Autodesk Fusion 360 part; units mm, degrees
(part 2 of 3)
sketch "motor_base_geometry" plane through (0, 0, 0) normal (0, 1, 0) x (1, 0, 0)
  line L0 (0, 120) -> (0, 140)
  line L1 (0, -20) -> (0, 0)
  line L2 (0, 40) -> (0, 60)
  line L3 (0, 100) -> (0, 120)
  line L4 (0, 20) -> (0, 40)
  line L5 (0, 0) -> (0, 20)
  line L6 (0, -40) -> (0, -20)
  line L7 (0, -80) -> (0, -60)
  line L8 (5, -200) -> (5, -220)
  line L9 (5, -180) -> (5, -200)
  line L10 (5, -340) -> (5, -360)
  line L11 (0, -380) -> (0, -360)
  line L12 (5, -440) -> (5, -460)
  line L13 (0, -200) -> (0, -180)
  line L14 (5, -80) -> (5, -100)
  line L15 (6, -520) -> (6, 520)
  line L16 (5, 520) -> (5, 500)
  line L17 (0, -400) -> (0, -380)
  line L18 (5, 380) -> (5, 360)
  line L19 (0, -100) -> (0, -80)
  line L20 (0, -220) -> (0, -200)
  line L21 (5, 0) -> (5, -20)
  line L22 (5, -100) -> (5, -120)
  line L23 (0, -180) -> (0, -160)
  line L24 (5, 360) -> (5, 340)
  line L25 (0, -624) -> (0, -520)
  line L26 (5, -480) -> (5, -500)
  line L27 (5, 500) -> (5, 480)
  line L28 (0, -520) -> (5, -520)
  line L29 (0, -120) -> (0, -100)
  line L30 (0, -440) -> (0, -420)
  line L31 (0, -260) -> (0, -240)
  line L32 (5, -60) -> (5, -80)
  line L33 (5, 20) -> (5, 0)
  line L34 (5, -40) -> (5, -60)
  line L35 (5, 120) -> (5, 100)
  line L36 (5, 440) -> (5, 420)
  line L37 (5, 240) -> (5, 220)
  line L38 (6, 520) -> (5, 520)
  line L39 (5, -400) -> (5, -420)
  line L40 (0, -500) -> (0, -480)
  line L41 (5, -240) -> (5, -260)
  line L42 (5, 100) -> (5, 80)
  line L43 (5, 300) -> (5, 280)
  line L44 (5, -420) -> (5, -440)
  line L45 (5, -20) -> (5, -40)
  line L46 (0, -420) -> (0, -400)
  line L47 (0, 520) -> (0, 624)
  line L48 (0, -340) -> (0, -320)
  line L49 (5, -260) -> (5, -280)
  line L50 (0, -140) -> (0, -120)
  line L51 (5, 280) -> (5, 260)
  line L52 (0, -480) -> (0, -460)
  line L53 (5, 60) -> (5, 40)
  line L54 (5, -160) -> (5, -180)
  line L55 (5, 160) -> (5, 140)
  line L56 (5, 180) -> (5, 160)
  line L57 (5, 200) -> (5, 180)
  line L58 (5, 40) -> (5, 20)
  line L59 (5, 140) -> (5, 120)
  line L60 (0, 460) -> (0, 480)
  line L61 (26.7, -624) -> (0, -624)
  line L62 (0, 480) -> (0, 500)
  line L63 (5, 260) -> (5, 240)
  line L64 (5, 420) -> (5, 400)
  line L65 (5, 80) -> (5, 60)
  line L66 (5, 220) -> (5, 200)
  line L67 (5, -520) -> (6, -520)
  line L68 (5, 320) -> (5, 300)
  line L69 (5, 460) -> (5, 440)
  line L70 (5, 400) -> (5, 380)
  line L71 (5, 480) -> (5, 460)
  line L72 (5, 340) -> (5, 320)
  line L73 (0, -160) -> (0, -140)
  line L74 (5, -360) -> (5, -380)
  line L75 (0, -320) -> (0, -300)
  line L76 (5, -380) -> (5, -400)
  line L77 (5, -500) -> (0, -500)
  line L78 (0, -360) -> (0, -340)
  line L79 (5, -300) -> (5, -320)
  line L80 (5, -140) -> (5, -160)
  line L81 (0, -300) -> (0, -280)
  line L82 (0, -240) -> (0, -220)
  line L83 (5, -120) -> (5, -140)
  line L84 (26.7, 624) -> (26.7, -624)
  line L85 (0, 320) -> (0, 340)
  line L86 (0, 420) -> (0, 440)
  line L87 (0, -280) -> (0, -260)
  line L88 (5, -220) -> (5, -240)
  line L89 (0, -460) -> (0, -440)
  line L90 (5, -320) -> (5, -340)
  line L91 (5, -280) -> (5, -300)
  line L92 (5, -460) -> (5, -480)
  line L93 (0, 440) -> (0, 460)
  line L94 (0, 360) -> (0, 380)
  line L95 (0, 624) -> (26.7, 624)
  line L96 (0, 340) -> (0, 360)
  line L97 (0, 300) -> (0, 320)
  line L98 (0, 260) -> (0, 280)
  line L99 (0, 220) -> (0, 240)
  line L100 (0, 240) -> (0, 260)
  line L101 (0, 180) -> (0, 200)
  line L102 (0, 160) -> (0, 180)
  line L103 (0, 280) -> (0, 300)
  line L104 (0, 200) -> (0, 220)
  line L105 (0, 140) -> (0, 160)
  line L106 (0, 80) -> (0, 100)
  line L107 (0, 60) -> (0, 80)
  line L108 (0, -60) -> (0, -40)
  line L109 (0, 400) -> (0, 420)
  line L110 (0, 500) -> (0, 520)
  line L111 (0, 380) -> (0, 400)
  line L112 (7.5, -30) -> (7.5, -25.1667)
  line L113 (7.5, -25.1667) -> (10.5, -25.1667)
  line L114 (10.5, -30) -> (7.5, -30)
  line L115 (10.5, -25.1667) -> (10.5, -30)
  line L116 (7.5, -18.3333) -> (10.5, -18.3333)
  line L117 (10.5, -23.1667) -> (7.5, -23.1667)
  line L118 (10.5, -18.3333) -> (10.5, -23.1667)
  line L119 (7.5, -23.1667) -> (7.5, -18.3333)
  line L120 (7.5, -16.3333) -> (7.5, -11.5)
  line L121 (10.5, -11.5) -> (10.5, -16.3333)
  line L122 (10.5, -16.3333) -> (7.5, -16.3333)
  line L123 (7.5, -11.5) -> (10.5, -11.5)
  line L124 (10.5, -9.5) -> (7.5, -9.5)
  line L125 (7.5, -9.5) -> (7.5, -4.6667)
  line L126 (7.5, -4.6667) -> (10.5, -4.6667)
  line L127 (10.5, -4.6667) -> (10.5, -9.5)
  line L128 (7.5, 2.1667) -> (10.5, 2.1667)
  line L129 (10.5, 2.1667) -> (10.5, -2.6667)
  line L130 (10.5, -2.6667) -> (7.5, -2.6667)
  line L131 (7.5, -2.6667) -> (7.5, 2.1667)
  line L132 (10.5, 9) -> (10.5, 4.1667)
  line L133 (7.5, 4.1667) -> (7.5, 9)
  line L134 (7.5, 9) -> (10.5, 9)
  line L135 (10.5, 4.1667) -> (7.5, 4.1667)
  line L136 (10.5, 11) -> (7.5, 11)
  line L137 (7.5, 11) -> (7.5, 15.8333)
  line L138 (10.5, 15.8333) -> (10.5, 11)
  line L139 (7.5, 15.8333) -> (10.5, 15.8333)
  line L140 (7.5, 22.6667) -> (10.5, 22.6667)
  line L141 (10.5, 22.6667) -> (10.5, 17.8333)
  line L142 (7.5, 17.8333) -> (7.5, 22.6667)
  line L143 (10.5, 17.8333) -> (7.5, 17.8333)
  line L144 (10.5, 24.6667) -> (7.5, 24.6667)
  line L145 (7.5, 24.6667) -> (7.5, 29.5)
  line L146 (7.5, 29.5) -> (10.5, 29.5)
  line L147 (10.5, 29.5) -> (10.5, 24.6667)
  line L148 (10.5, 31.5) -> (7.5, 31.5)
  line L149 (7.5, 36.3333) -> (10.5, 36.3333)
  line L150 (7.5, 31.5) -> (7.5, 36.3333)
  line L151 (10.5, 36.3333) -> (10.5, 31.5)
  line L152 (7.5, 38.3333) -> (7.5, 43.1667)
  line L153 (10.5, 43.1667) -> (10.5, 38.3333)
  line L154 (7.5, 43.1667) -> (10.5, 43.1667)
  line L155 (10.5, 38.3333) -> (7.5, 38.3333)
  line L156 (10.5, 45.1667) -> (7.5, 45.1667)
  line L157 (7.5, 50) -> (10.5, 50)
  line L158 (10.5, 50) -> (10.5, 45.1667)
  line L159 (7.5, 45.1667) -> (7.5, 50)
  line L160 (10.5, 45.1667) -> (10.5, 43.1667)
  line L161 (10.5, 38.3333) -> (10.5, 36.3333)
  line L162 (10.5, 31.5) -> (10.5, 29.5)
  line L163 (10.5, 24.6667) -> (10.5, 22.6667)
  line L164 (10.5, 17.8333) -> (10.5, 15.8333)
  line L165 (10.5, 4.1667) -> (10.5, 2.1667)
  line L166 (10.5, -2.6667) -> (10.5, -4.6667)
  line L167 (10.5, -9.5) -> (10.5, -11.5)
  line L168 (10.5, -16.3333) -> (10.5, -18.3333)
  line L169 (10.5, -23.1667) -> (10.5, -25.1667)
  line L170 (17.8, 45.25) -> (12.3, 45.25)
  line L171 (17.8, 47.25) -> (12.3, 47.25)
  line L172 (12.3, 44.75) -> (17.8, 44.75)
  line L173 (17.8, 39.25) -> (12.3, 39.25)
  line L174 (17.8, 37.25) -> (12.3, 37.25)
  line L175 (17.8, 30.75) -> (17.8, 31.25)
  line L176 (17.8, 26.75) -> (17.8, 27.25)
  line L177 (17.8, 40.75) -> (17.8, 41.25)
  line L178 (12.3, 35.25) -> (12.3, 36.75)
  line L179 (17.8, 36.75) -> (17.8, 37.25)
  line L180 (17.8, 28.75) -> (17.8, 29.25)
  line L181 (12.3, 28.75) -> (17.8, 28.75)
  line L182 (12.3, 40.75) -> (17.8, 40.75)
  line L183 (12.3, 38.75) -> (17.8, 38.75)
  line L184 (17.8, 41.25) -> (12.3, 41.25)
  line L185 (12.3, 33.25) -> (12.3, 34.75)
  line L186 (17.8, 29.25) -> (12.3, 29.25)
  line L187 (17.8, 49.25) -> (12.3, 49.25)
  line L188 (17.8, 25.25) -> (12.3, 25.25)
  line L189 (17.8, 35.25) -> (12.3, 35.25)
  line L190 (17.8, 38.75) -> (17.8, 39.25)
  line L191 (12.3, 39.25) -> (12.3, 40.75)
  line L192 (17.8, 34.75) -> (17.8, 35.25)
  line L193 (12.3, 42.75) -> (17.8, 42.75)
  line L194 (12.3, 27.25) -> (12.3, 28.75)
  line L195 (17.8, 48.75) -> (17.8, 49.25)
  line L196 (12.3, 36.75) -> (17.8, 36.75)
  line L197 (17.8, 43.25) -> (12.3, 43.25)
  line L198 (17.8, 46.75) -> (17.8, 47.25)
  line L199 (12.3, 49.25) -> (12.3, 50.75)
  line L200 (12.3, 47.25) -> (12.3, 48.75)
  line L201 (12.3, 30.75) -> (17.8, 30.75)
  line L202 (12.3, 29.25) -> (12.3, 30.75)
  line L203 (12.3, 37.25) -> (12.3, 38.75)
  line L204 (12.3, 43.25) -> (12.3, 44.75)
  line L205 (17.8, 50.75) -> (17.8, 51.25)
  line L206 (12.3, 50.75) -> (17.8, 50.75)
  line L207 (12.3, 25.25) -> (12.3, 26.75)
  line L208 (12.3, 46.75) -> (17.8, 46.75)
  line L209 (17.8, 31.25) -> (12.3, 31.25)
  line L210 (17.8, -9.25) -> (17.8, -8.75)
  line L211 (12.3, 3.25) -> (12.3, 4.75)
  line L212 (12.3, 24.75) -> (17.8, 24.75)
  line L213 (17.8, -7.25) -> (17.8, -6.75)
  line L214 (17.8, 12.75) -> (17.8, 13.25)
  line L215 (17.8, 16.75) -> (17.8, 17.25)
  line L216 (17.8, 15.25) -> (12.3, 15.25)
  line L217 (12.3, 2.75) -> (17.8, 2.75)
  line L218 (17.8, -6.75) -> (12.3, -6.75)
  line L219 (17.8, -2.75) -> (12.3, -2.75)
  line L220 (12.3, 10.75) -> (17.8, 10.75)
  line L221 (17.8, 21.25) -> (12.3, 21.25)
  line L222 (12.3, 22.75) -> (17.8, 22.75)
  line L223 (12.3, 1.25) -> (12.3, 2.75)
  line L224 (17.8, 32.75) -> (17.8, 33.25)
  line L225 (12.3, 41.25) -> (12.3, 42.75)
  line L226 (17.8, 24.75) -> (17.8, 25.25)
  line L227 (17.8, 19.25) -> (12.3, 19.25)
  line L228 (12.3, 26.75) -> (17.8, 26.75)
  line L229 (12.3, 45.25) -> (12.3, 46.75)
  line L230 (17.8, 6.75) -> (17.8, 7.25)
  line L231 (12.3, 48.75) -> (17.8, 48.75)
  line L232 (17.8, 51.25) -> (17.8, 51.4522)
  line L233 (11.5, 51.4522) -> (11.5, 51.25)
  line L234 (11.5, 51.25) -> (11.5, 50)
  line L235 (17.8, 8.75) -> (17.8, 9.25)
  line L236 (12.3, 31.25) -> (12.3, 32.75)
  line L237 (17.8, 33.25) -> (12.3, 33.25)
  line L238 (12.3, -1.25) -> (17.8, -1.25)
  line L239 (17.8, 27.25) -> (12.3, 27.25)
  line L240 (17.8, -17.25) -> (17.8, -16.75)
  line L241 (17.8, 51.4522) -> (11.5, 51.4522)
  line L242 (17.8, -31.25) -> (17.8, -30.75)
  line L243 (17.8, -26.75) -> (12.3, -26.75)
  line L244 (12.3, 32.75) -> (17.8, 32.75)
  line L245 (17.8, 9.25) -> (12.3, 9.25)
  line L246 (12.3, -3.25) -> (17.8, -3.25)
  line L247 (17.8, 10.75) -> (17.8, 11.25)
  line L248 (12.3, 15.25) -> (12.3, 16.75)
  line L249 (12.3, -6.75) -> (12.3, -5.25)
  line L250 (12.3, 12.75) -> (17.8, 12.75)
  line L251 (12.3, 6.75) -> (17.8, 6.75)
  line L252 (17.8, 22.75) -> (17.8, 23.25)
  line L253 (17.8, -4.75) -> (12.3, -4.75)
  line L254 (12.3, -0.75) -> (12.3, 0.75)
  line L255 (11.5, 50) -> (11.5, -30)
  line L256 (17.8, -24.75) -> (12.3, -24.75)
  line L257 (17.8, -12.75) -> (12.3, -12.75)
  line L258 (17.8, -29.25) -> (17.8, -28.75)
  line L259 (17.8, -28.75) -> (12.3, -28.75)
  line L260 (17.8, -16.75) -> (12.3, -16.75)
  line L261 (12.3, -29.25) -> (17.8, -29.25)
  line L262 (12.3, -25.25) -> (17.8, -25.25)
  line L263 (12.3, -16.75) -> (12.3, -15.25)
  line L264 (17.8, -23.25) -> (17.8, -22.75)
  line L265 (17.8, 44.75) -> (17.8, 45.25)
  line L266 (17.8, -10.75) -> (12.3, -10.75)
  line L267 (9, -35) -> (6.5, -35)
  line L268 (12.3, -32.75) -> (12.3, -31.25)
  line L269 (12.3, -22.75) -> (12.3, -21.25)
  line L270 (12.3, -18.75) -> (12.3, -17.25)
  line L271 (17.8, -30.75) -> (12.3, -30.75)
  line L272 (12.3, -15.25) -> (17.8, -15.25)
  line L273 (17.8, -25.25) -> (17.8, -24.75)
  line L274 (17.8, -15.25) -> (17.8, -14.75)
  line L275 (12.3, -12.75) -> (12.3, -11.25)
  line L276 (10.7, -35) -> (9, -35)
  line L277 (17.8, -38) -> (17.8, -33.25)
  line L278 (12.3, -23.25) -> (17.8, -23.25)
  line L279 (17.8, -32.75) -> (12.3, -32.75)
  line L280 (17.8, -21.25) -> (17.8, -20.75)
  line L281 (6.5, -35) -> (6.5, -38)
  line L282 (12.3, -28.75) -> (12.3, -27.25)
  line L283 (12.3, -27.25) -> (17.8, -27.25)
  line L284 (17.8, -11.25) -> (17.8, -10.75)
  line L285 (12.3, 34.75) -> (17.8, 34.75)
  line L286 (12.3, -14.75) -> (12.3, -13.25)
  line L287 (12.3, -21.25) -> (17.8, -21.25)
  line L288 (11.5, -30) -> (11.5, -35)
  line L289 (12.3, -19.25) -> (17.8, -19.25)
  line L290 (17.8, -14.75) -> (12.3, -14.75)
  line L291 (17.8, -18.75) -> (12.3, -18.75)
  line L292 (12.3, 13.25) -> (12.3, 14.75)
  line L293 (12.3, 11.25) -> (12.3, 12.75)
  line L294 (12.3, -4.75) -> (12.3, -3.25)
  line L295 (17.8, 0.75) -> (17.8, 1.25)
  line L296 (12.3, 16.75) -> (17.8, 16.75)
  line L297 (17.8, 11.25) -> (12.3, 11.25)
  line L298 (17.8, -13.25) -> (17.8, -12.75)
  line L299 (17.8, -22.75) -> (12.3, -22.75)
  line L300 (17.8, -33.25) -> (17.8, -32.75)
  line L301 (11.5, -35) -> (10.7, -35)
  line L302 (12.3, -8.75) -> (12.3, -7.25)
  line L303 (12.3, -17.25) -> (17.8, -17.25)
  line L304 (12.3, -11.25) -> (17.8, -11.25)
  line L305 (17.8, 42.75) -> (17.8, 43.25)
  line L306 (6.5, -38) -> (17.8, -38)
  line L307 (12.3, -20.75) -> (12.3, -19.25)
  line L308 (17.8, -27.25) -> (17.8, -26.75)
  line L309 (17.8, -19.25) -> (17.8, -18.75)
  line L310 (12.3, -31.25) -> (17.8, -31.25)
  line L311 (17.8, -20.75) -> (12.3, -20.75)
  line L312 (12.3, -9.25) -> (17.8, -9.25)
  line L313 (12.3, -30.75) -> (12.3, -29.25)
  line L314 (12.3, -13.25) -> (17.8, -13.25)
  line L315 (17.8, -8.75) -> (12.3, -8.75)
  line L316 (12.3, -7.25) -> (17.8, -7.25)
  line L317 (12.3, -26.75) -> (12.3, -25.25)
  line L318 (12.3, -24.75) -> (12.3, -23.25)
  line L319 (12.3, -10.75) -> (12.3, -9.25)
  line L320 (12.3, 17.25) -> (12.3, 18.75)
  line L321 (17.8, 17.25) -> (12.3, 17.25)
  line L322 (12.3, 20.75) -> (17.8, 20.75)
  line L323 (17.8, -1.25) -> (17.8, -0.75)
  line L324 (17.8, 13.25) -> (12.3, 13.25)
  line L325 (17.8, -0.75) -> (12.3, -0.75)
  line L326 (17.8, -5.25) -> (17.8, -4.75)
  line L327 (17.8, 3.25) -> (12.3, 3.25)
  line L328 (17.8, 5.25) -> (12.3, 5.25)
  line L329 (17.8, 2.75) -> (17.8, 3.25)
  line L330 (17.8, 20.75) -> (17.8, 21.25)
  line L331 (17.8, 1.25) -> (12.3, 1.25)
  line L332 (12.3, 23.25) -> (12.3, 24.75)
  line L333 (12.3, 4.75) -> (17.8, 4.75)
  line L334 (12.3, 7.25) -> (12.3, 8.75)
  line L335 (12.3, 18.75) -> (17.8, 18.75)
  line L336 (12.3, -2.75) -> (12.3, -1.25)
  line L337 (17.8, 18.75) -> (17.8, 19.25)
  line L338 (12.3, 0.75) -> (17.8, 0.75)
  line L339 (17.8, 4.75) -> (17.8, 5.25)
  line L340 (12.3, 21.25) -> (12.3, 22.75)
  line L341 (17.8, 14.75) -> (17.8, 15.25)
  line L342 (17.8, -3.25) -> (17.8, -2.75)
  line L343 (17.8, 23.25) -> (12.3, 23.25)
  line L344 (12.3, 14.75) -> (17.8, 14.75)
  line L345 (12.3, -5.25) -> (17.8, -5.25)
  line L346 (12.3, 9.25) -> (12.3, 10.75)
  line L347 (12.3, 19.25) -> (12.3, 20.75)
  line L348 (12.3, 5.25) -> (12.3, 6.75)
  line L349 (12.3, 8.75) -> (17.8, 8.75)
  line L350 (17.8, 7.25) -> (12.3, 7.25)
  line L351 (6.5, -35) -> (6.5, 55)
  line L352 (0, -520) -> (0, -500)
  line L353 (5, -500) -> (5, -520)
  line L354 (0, -480) -> (5, -480)
  line L355 (0, -460) -> (5, -460)
  line L356 (0, -440) -> (5, -440)
  line L357 (0, -420) -> (5, -420)
  line L358 (0, -400) -> (5, -400)
  line L359 (0, -380) -> (5, -380)
  line L360 (0, -360) -> (5, -360)
  line L361 (0, -340) -> (5, -340)
  line L362 (0, -320) -> (5, -320)
  line L363 (0, -300) -> (5, -300)
  line L364 (0, -280) -> (5, -280)
  line L365 (0, -260) -> (5, -260)
  line L366 (0, -240) -> (5, -240)
  line L367 (0, -220) -> (5, -220)
  line L368 (0, -200) -> (5, -200)
  line L369 (0, -180) -> (5, -180)
  line L370 (0, -160) -> (5, -160)
  line L371 (0, -140) -> (5, -140)
  line L372 (0, -120) -> (5, -120)
  line L373 (0, -100) -> (5, -100)
  line L374 (0, -80) -> (5, -80)
  line L375 (0, -60) -> (5, -60)
  line L376 (0, -40) -> (5, -40)
  line L377 (0, -20) -> (5, -20)
  line L378 (0, 0) -> (5, 0)
  line L379 (0, 20) -> (5, 20)
  line L380 (0, 40) -> (5, 40)
  line L381 (0, 60) -> (5, 60)
  line L382 (0, 80) -> (5, 80)
  line L383 (0, 100) -> (5, 100)
  line L384 (0, 120) -> (5, 120)
  line L385 (0, 140) -> (5, 140)
  line L386 (0, 160) -> (5, 160)
  line L387 (0, 180) -> (5, 180)
  line L388 (0, 200) -> (5, 200)
  line L389 (0, 220) -> (5, 220)
  line L390 (0, 240) -> (5, 240)
  line L391 (0, 260) -> (5, 260)
  line L392 (0, 280) -> (5, 280)
  line L393 (0, 300) -> (5, 300)
  line L394 (0, 320) -> (5, 320)
  line L395 (0, 340) -> (5, 340)
  line L396 (0, 360) -> (5, 360)
  line L397 (0, 380) -> (5, 380)
  line L398 (0, 400) -> (5, 400)
  line L399 (0, 420) -> (5, 420)
  line L400 (0, 440) -> (5, 440)
  line L401 (0, 460) -> (5, 460)
  line L402 (0, 480) -> (5, 480)
  line L403 (0, 500) -> (5, 500)
  line L404 (0, 520) -> (5, 520)
  line L405 (17.8, -33.25) -> (12.3, -33.25)
  line L406 (12.3, -33.25) -> (12.3, -34.75)
  line L407 (10.5, 11) -> (10.5, 9)
  line L408 (12.3, -34.75) -> (12.3, -35)
  line L409 (12.3, -35) -> (11.5, -35)
  line L410 (9, -35) -> (9.1, -35)
  line L411 (12.3, -35) -> (12.4, -35)
  line L412 (12.4, -35) -> (12.4, -33.25)
  line L413 (10.5, 50) -> (11.4, 50)
  line L414 (11.4, 50) -> (11.4, 51.4522)
  line L415 (11.4, 51.4522) -> (11.5, 51.4522)
  line L416 (6.5, 55) -> (17.8, 55)
  line L417 (17.8, 55) -> (17.8, 51.4522)
  line L418 (10.5, -30) -> (10.7, -30)
  line L419 (10.7, -30) -> (10.7, -33)
  line L420 (10.7, -33) -> (10.7, -35)
revolve "Revolve1" add sketch "motor_base_geometry" angle 360 about axis through (0, 0, 20) along (0, 0, -1) contours L112 L113 L114 L115
chamfer "Chamfer1" distance 0.2 angle 45 4 edges at (-9.7894, -3.797, 30) (-9.7894, -3.797, 25.1667) (-6.9925, -2.7121, 30) (-6.9925, -2.7121, 25.1667)
named bodies: "coil"

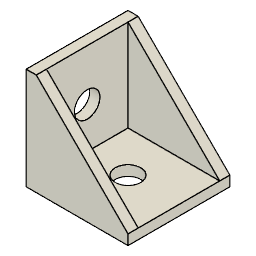
design "Aluminium connections"
Autodesk Fusion 360 part; units mm, degrees
sketch "Base & hole" plane through (0, 0, 0) normal (0, 1, 0) x (1, 0, 0)
  line L0 (0, 0) -> (20, 0)
  line L1 (20, 0) -> (20, 20)
  line L2 (20, 20) -> (0, 20)
  line L3 (0, 20) -> (0, 0)
  circle A0 centre (10, 10) radius 2.5
  dimension "d1" = 20
  dimension "d2" = 20
  dimension "d3" = 5
  constraint horizontal L0
  constraint vertical L1
  constraint horizontal L2
  constraint vertical L3
  constraint coincident L0.start L3.end
  measures "d1" distance of L0.start L0.end
  measures "d2" distance of L0.start L2.end
  measures "d3" diameter of A0
extrude "Extrude1" add sketch "Base & hole" along normal blind 20
sketch "Top" plane through (0, 20, 0) normal (0, 1, 0) x (-1, 0, 0)
  circle A0 centre (-10, -10) radius 2.5
  line L0 (0, -20) -> (0, 0)
  line L1 (0, 0) -> (-20, 0)
  line L2 (-20, 0) -> (-20, -20)
  line L3 (-20, -20) -> (0, -20)
  line L4 (-20, -20) -> (-20, -18) construction
  line L5 (-20, -18) -> (-2, -18)
  line L6 (-2, -18) -> (-2, -2)
  line L7 (-2, -2) -> (-20, -2)
  dimension "d6" = 2
  dimension "d7" = 18
  dimension "d8" = 16
  constraint coincident L2.end L3.start
  constraint perpendicular L3 L4
  constraint perpendicular L0 L5
  constraint perpendicular L3 L6
  constraint coincident L2 L7.end
  constraint perpendicular L2 L7
  measures "d6" distance of L2.end L4.end
  measures "d7" distance of L4.end L5.end
  measures "d8" distance of L5.end L6.end
extrude "Extrude2" cut sketch "Top" against normal blind 18 contours L2 L5 L6 L7
sketch "Side removal" plane through (0, 0, 0) normal (0, 0, 1) x (1, 0, 0)
  line L0 (0, 0) -> (20, 0)
  line L1 (20, 0) -> (20, 20)
  line L2 (20, 20) -> (0, 20)
  line L3 (0, 20) -> (0, 0)
  line L4 (0, 20) -> (2, 20)
  line L5 (20, 0) -> (20, 2)
  line L6 (20, 2) -> (2, 20)
  dimension "d11" = 2
  dimension "d12" = 2
  constraint coincident L2.end L3.start
  constraint perpendicular L3 L4
  constraint coincident L0.end L1.start
  constraint perpendicular L0 L5
  measures "d11" distance of L2.end L4.end
  measures "d12" distance of L0.end L5.end
extrude "Extrude3" cut sketch "Side removal" against normal blind 30 contours L1 L2 L6
sketch "side hole" plane through (0, 0, 0) normal (-1, 0, 0) x (0, 0, 1)
  line L0 (-20, 0) -> (0, 0)
  line L1 (0, 0) -> (0, 20)
  line L2 (0, 20) -> (-20, 20)
  line L3 (-20, 20) -> (-20, 0)
  circle A0 centre (-10, 10) radius 2.5
  dimension "d15" = 5
  measures "d15" diameter of A0
extrude "Extrude4" cut sketch "side hole" against normal blind 5 contours A0

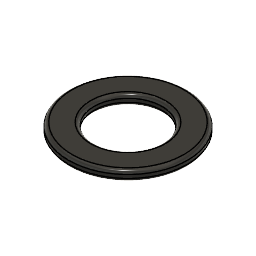
design "m2 by 0.3 spacer"
Autodesk Fusion 360 part; units mm, degrees
sketch "Sketch1" plane through (0, 0, 0) normal (0, 1, 0) x (1, 0, 0)
  circle A0 centre (0, 0) radius 1
  circle A1 centre (0, 0) radius 1.75
  dimension "d1" = 2
  dimension "d2" = 3.5
  constraint coincident A0.centre A1.centre
  measures "d1" diameter of A0
  measures "d2" diameter of A1
extrude "Extrude1" add sketch "Sketch1" along normal blind 0.3
fillet "Fillet1" radius 0.1 4 edges at (-0.9323, 0.3, -0.3616) (-0.9323, 0, -0.3616) (-1.6316, 0.3, 0.6328) (-1.6316, 0, 0.6328)

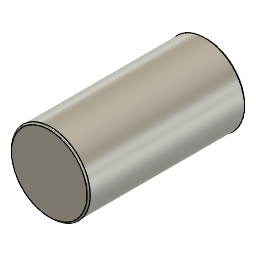
design "15mm by 20mm axial magnet"
Autodesk Fusion 360 part; units mm, degrees
sketch "Sketch1" plane through (0, 0, 0) normal (0, 0, 1) x (1, 0, 0)
  circle A0 centre (0, 0) radius 5
  dimension "d1" = 10
  constraint coincident A0.centre origin
  measures "d1" diameter of A0
extrude "Extrude1" add sketch "Sketch1" along normal blind 20
fillet "Fillet1" radius 0.2 2 edges at (-4.6616, -1.8081, 20) (-4.6616, -1.8081, 0)

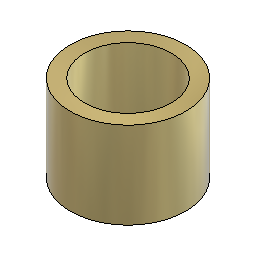
design "M3 x 3 Insert"
Autodesk Fusion 360 part; units mm, degrees
sketch "Sketch1" plane through (0, 0, 0) normal (0, 1, 0) x (1, 0, 0)
  circle A0 centre (0, 0) radius 1.5
  circle A1 centre (0, 0) radius 2
  dimension "d1" = 3
  dimension "d2" = 4
  constraint coincident A0.centre A1.centre
  measures "d1" diameter of A0
  measures "d2" diameter of A1
extrude "Extrude1" add sketch "Sketch1" along normal blind 5
extrude "Extrude2" cut 1 faces at (1.8259, 5, 0.0994) along direction (0, -1, 0) blind 2

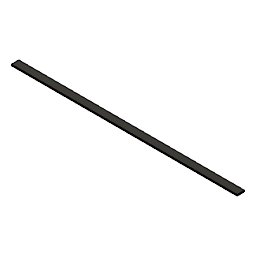
design "linear scale"
Autodesk Fusion 360 part; units mm, degrees
sketch "base" plane through (0, 0, 0) normal (0, 1, 0) x (1, 0, 0)
  line L0 (0, 0) -> (-300, 0)
  line L1 (-300, 0) -> (-300, 10)
  line L2 (-300, 10) -> (0, 10)
  line L3 (0, 10) -> (0, 0)
  dimension "d1" = 300
  dimension "d2" = 10
  constraint coincident L0.start L3.end
  constraint horizontal L0
  constraint perpendicular L0 L1
  constraint perpendicular L1 L2
  constraint perpendicular L0 L3
  measures "d1" distance of L0.start L0.end
  measures "d2" distance of L0.end L1.end
extrude "Extrude1" add sketch "base" along normal blind 1.4
named bodies: "main"

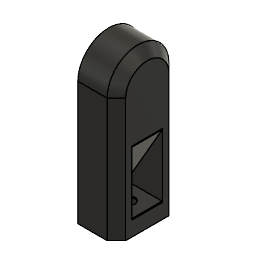
design "stator_holders"
Autodesk Fusion 360 part; units mm, degrees
sketch "Base" plane through (0, 0, 0) normal (1, 0, 0) x (0, 0, -1)
  circle A0 centre (0, 0) radius 6.1
  circle A1 centre (0, 0) radius 10 construction
  line L0 (0, 0) -> (-10, 0) construction
  line L1 (0, 0) -> (0, -40) construction
  line L2 (0, -40) -> (-10, -40)
  line L3 (-10, -40) -> (-10, 0)
  line L4 (10, -40) -> (10, 0)
  line L5 (0, -40) -> (10, -40)
  line L6 (0, 0) -> (0, 10) construction
  arc A2 (10, 0) -> (-10, 0) centre (0, 0) ccw
  dimension "d1" = 12.2
  dimension "d2" = 20
  dimension "d3" = 40
  dimension "d4" = 10
  constraint coincident A0.centre A1.centre
  constraint concentric A0 A1
  constraint coincident A1 L0.end
  constraint horizontal L0
  constraint perpendicular L0 L1
  constraint perpendicular L1 L2
  constraint symmetric L0.end L1 L4.end
  constraint symmetric L2.start L1 L5.start
  constraint symmetric L1 L2.end L4.start
  constraint coincident A1 L6.end
  constraint perpendicular L0 L6
  constraint coincident L6.end A2
  measures "d1" diameter of A0
  measures "d2" diameter of A1
  measures "d3" distance of A0.centre L1.end
  measures "d4" distance of L1.end L2.end
extrude "Extrude1" add sketch "Base" along normal blind 12.5 contours A0 | L2 L3 L4 L5 A2
extrude "Extrude2" cut sketch "Base" along normal blind 10 contours A0
chamfer "Chamfer1" distance 3 angle 45 3 edges at (12.5, 10, 0) (12.5, -20, 10) (12.5, -20, -10)
ref_plane "WorkPlane1" through (6.25, -20, 0) normal (0, 0, -1) x (0, 1, 0)
sketch "Bolt" plane through (0, 0, 0) normal (0, 0, -1) x (0, 1, 0)
  line L0 (0, 0) -> (-30, 0) construction
  line L1 (-30, 0) -> (-30, 12.5) construction
  line L2 (-30, 12.5) -> (0, 12.5) construction
  line L3 (0, 12.5) -> (0, 0) construction
  line L4 (-30, 12.5) -> (-35, 12.5) construction
  line L5 (-35, 12.5) -> (-35, 0) construction
  line L6 (-35, 12.5) -> (-35, 2.5)
  line L7 (-35, 2.5) -> (-32, 2.5)
  line L8 (-32, 2.5) -> (-14.6795, 12.5)
  line L9 (-35, 12.5) -> (-14.6795, 12.5)
  dimension "d11" = 12.5
  dimension "d12" = 10
  dimension "d13" = 20
  constraint horizontal L0
  constraint vertical L1
  constraint horizontal L2
  constraint vertical L3
  constraint coincident L0.start L3.end
  constraint coincident L2 L4.end
  constraint coincident L0 L5.end
  constraint perpendicular L0 L5
  constraint perpendicular L2 L6
  constraint perpendicular L6 L7
  constraint coincident L2 L8.end
  measures "d11" distance of L0.start L2.end
  measures "d12" distance of L4.end L6.end
  measures "d13" distance of L7.end L8.end
extrude "Extrude3" cut sketch "Bolt" along normal blind 5
extrude "Extrude4" cut 1 faces at (9.1667, -27.2265, 0) along direction (0, 0, 1) blind 5
sketch "Sketch3" plane through (0, -35, 0) normal (0, 1, 0) x (-1, 0, 0)
  line L0 (-12.5, 5) -> (-12.5, -5)
  line L1 (-12.5, -5) -> (-2.5, -5)
  line L2 (-2.5, -5) -> (-2.5, 5)
  line L3 (-2.5, 5) -> (-12.5, 5)
  line L4 (-12.5, 5) -> (-2.5, 5)
  line L5 (-2.5, 5) -> (-2.5, -5)
  line L6 (-2.5, -5) -> (-12.5, -5)
  line L7 (-12.5, -5) -> (-12.5, 5)
  circle A0 centre (-7, 0) radius 1.5
  dimension "d18" = 3
  constraint horizontal L4
  constraint vertical L5
  constraint horizontal L6
  constraint vertical L7
  constraint coincident L1.end L2.start
  constraint coincident L0.start L3.end
  measures "d18" diameter of A0
extrude "Extrude5" cut sketch "Sketch3" against normal blind 6 contours A0
chamfer "Chamfer2" distance 0.2 angle 45 1 edges at (8.3985, -35, 0.5424)
chamfer "Chamfer3" distance 0.2 angle 45 4 edges at (2.5, -35, 0) (2.5, -32, 0) (12.5, -14.6795, 0) (12.5, -35, 0)
chamfer "Chamfer4" distance 0.3 angle 45 1 edges at (0, -2.2059, 5.6872)

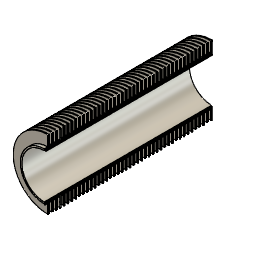
design "heat_sink"
Autodesk Fusion 360 part; units mm, degrees
sketch "motor_base_geometry" plane through (0, 0, 0) normal (0, 1, 0) x (1, 0, 0)
  line L0 (0, -624) -> (0, -520)
  line L1 (0, 624) -> (26.7, 624)
  line L2 (26.7, 624) -> (26.7, -624)
  line L3 (26.7, -624) -> (0, -624)
  line L4 (0, 520) -> (0, 624)
  line L5 (7.5, -30) -> (7.5, -25.1667)
  line L6 (7.5, -25.1667) -> (10.5, -25.1667)
  line L7 (10.5, -30) -> (7.5, -30)
  line L8 (7.5, -23.1667) -> (7.5, -18.3333)
  line L9 (7.5, -18.3333) -> (10.5, -18.3333)
  line L10 (10.5, -23.1667) -> (7.5, -23.1667)
  line L11 (7.5, -16.3333) -> (7.5, -11.5)
  line L12 (7.5, -11.5) -> (10.5, -11.5)
  line L13 (10.5, -16.3333) -> (7.5, -16.3333)
  line L14 (7.5, -9.5) -> (7.5, -4.6667)
  line L15 (7.5, -4.6667) -> (10.5, -4.6667)
  line L16 (10.5, -9.5) -> (7.5, -9.5)
  line L17 (7.5, -2.6667) -> (7.5, 2.1667)
  line L18 (7.5, 2.1667) -> (10.5, 2.1667)
  line L19 (10.5, -2.6667) -> (7.5, -2.6667)
  line L20 (7.5, 4.1667) -> (7.5, 9)
  line L21 (7.5, 9) -> (10.5, 9)
  line L22 (10.5, 4.1667) -> (7.5, 4.1667)
  line L23 (7.5, 11) -> (7.5, 15.8333)
  line L24 (7.5, 15.8333) -> (10.5, 15.8333)
  line L25 (10.5, 11) -> (7.5, 11)
  line L26 (7.5, 17.8333) -> (7.5, 22.6667)
  line L27 (7.5, 22.6667) -> (10.5, 22.6667)
  line L28 (10.5, 17.8333) -> (7.5, 17.8333)
  line L29 (7.5, 24.6667) -> (7.5, 29.5)
  line L30 (7.5, 29.5) -> (10.5, 29.5)
  line L31 (10.5, 24.6667) -> (7.5, 24.6667)
  line L32 (7.5, 31.5) -> (7.5, 36.3333)
  line L33 (7.5, 36.3333) -> (10.5, 36.3333)
  line L34 (10.5, 31.5) -> (7.5, 31.5)
  line L35 (7.5, 38.3333) -> (7.5, 43.1667)
  line L36 (7.5, 43.1667) -> (10.5, 43.1667)
  line L37 (10.5, 38.3333) -> (7.5, 38.3333)
  line L38 (7.5, 45.1667) -> (7.5, 50)
  line L39 (7.5, 50) -> (10.5, 50)
  line L40 (10.5, 45.1667) -> (7.5, 45.1667)
  line L41 (10.5, 45.1667) -> (10.5, 43.1667)
  line L42 (10.5, 38.3333) -> (10.5, 36.3333)
  line L43 (10.5, 31.5) -> (10.5, 29.5)
  line L44 (10.5, 24.6667) -> (10.5, 22.6667)
  line L45 (10.5, 17.8333) -> (10.5, 15.8333)
  line L46 (10.5, 4.1667) -> (10.5, 2.1667)
  line L47 (10.5, -2.6667) -> (10.5, -4.6667)
  line L48 (10.5, -9.5) -> (10.5, -11.5)
  line L49 (10.5, -16.3333) -> (10.5, -18.3333)
  line L50 (10.5, -23.1667) -> (10.5, -25.1667)
  line L51 (11.5, -30) -> (11.5, -35)
  line L52 (6.5, -35) -> (6.5, 55)
  line L53 (10.5, -25.1667) -> (10.5, -30)
  line L54 (10.5, -18.3333) -> (10.5, -23.1667)
  line L55 (10.5, -11.5) -> (10.5, -16.3333)
  line L56 (10.5, -4.6667) -> (10.5, -9.5)
  line L57 (10.5, 2.1667) -> (10.5, -2.6667)
  line L58 (10.5, 9) -> (10.5, 4.1667)
  line L59 (10.5, 15.8333) -> (10.5, 11)
  line L60 (10.5, 22.6667) -> (10.5, 17.8333)
  line L61 (10.5, 29.5) -> (10.5, 24.6667)
  line L62 (10.5, 36.3333) -> (10.5, 31.5)
  line L63 (10.5, 43.1667) -> (10.5, 38.3333)
  line L64 (10.5, 50) -> (10.5, 45.1667)
  line L65 (0, -520) -> (0, -500)
  line L66 (0, -500) -> (0, -480)
  line L67 (0, -500) -> (5, -500)
  line L68 (5, -500) -> (5, -520)
  line L69 (5, -520) -> (0, -520)
  line L70 (0, -480) -> (0, -460)
  line L71 (0, -480) -> (5, -480)
  line L72 (5, -480) -> (5, -500)
  line L73 (0, -460) -> (0, -440)
  line L74 (0, -460) -> (5, -460)
  line L75 (5, -460) -> (5, -480)
  line L76 (0, -440) -> (0, -420)
  line L77 (0, -440) -> (5, -440)
  line L78 (5, -440) -> (5, -460)
  line L79 (0, -420) -> (0, -400)
  line L80 (0, -420) -> (5, -420)
  line L81 (5, -420) -> (5, -440)
  line L82 (0, -400) -> (0, -380)
  line L83 (0, -400) -> (5, -400)
  line L84 (5, -400) -> (5, -420)
  line L85 (0, -380) -> (0, -360)
  line L86 (0, -380) -> (5, -380)
  line L87 (5, -380) -> (5, -400)
  line L88 (0, -360) -> (0, -340)
  line L89 (0, -360) -> (5, -360)
  line L90 (5, -360) -> (5, -380)
  line L91 (0, -340) -> (0, -320)
  line L92 (0, -340) -> (5, -340)
  line L93 (5, -340) -> (5, -360)
  line L94 (0, -320) -> (0, -300)
  line L95 (0, -320) -> (5, -320)
  line L96 (5, -320) -> (5, -340)
  line L97 (0, -300) -> (0, -280)
  line L98 (0, -300) -> (5, -300)
  line L99 (5, -300) -> (5, -320)
  line L100 (0, -280) -> (0, -260)
  line L101 (0, -280) -> (5, -280)
  line L102 (5, -280) -> (5, -300)
  line L103 (0, -260) -> (0, -240)
  line L104 (0, -260) -> (5, -260)
  line L105 (5, -260) -> (5, -280)
  line L106 (0, -240) -> (0, -220)
  line L107 (0, -240) -> (5, -240)
  line L108 (5, -240) -> (5, -260)
  line L109 (0, -220) -> (0, -200)
  line L110 (0, -220) -> (5, -220)
  line L111 (5, -220) -> (5, -240)
  line L112 (0, -200) -> (0, -180)
  line L113 (0, -200) -> (5, -200)
  line L114 (5, -200) -> (5, -220)
  line L115 (0, -180) -> (0, -160)
  line L116 (0, -180) -> (5, -180)
  line L117 (5, -180) -> (5, -200)
  line L118 (0, -160) -> (0, -140)
  line L119 (0, -160) -> (5, -160)
  line L120 (5, -160) -> (5, -180)
  line L121 (0, -140) -> (0, -120)
  line L122 (0, -140) -> (5, -140)
  line L123 (5, -140) -> (5, -160)
  line L124 (0, -120) -> (0, -100)
  line L125 (0, -120) -> (5, -120)
  line L126 (5, -120) -> (5, -140)
  line L127 (0, -100) -> (0, -80)
  line L128 (0, -100) -> (5, -100)
  line L129 (5, -100) -> (5, -120)
  line L130 (0, -80) -> (0, -60)
  line L131 (0, -80) -> (5, -80)
  line L132 (5, -80) -> (5, -100)
  line L133 (0, -60) -> (0, -40)
  line L134 (0, -60) -> (5, -60)
  line L135 (5, -60) -> (5, -80)
  line L136 (0, -40) -> (0, -20)
  line L137 (0, -40) -> (5, -40)
  line L138 (5, -40) -> (5, -60)
  line L139 (0, -20) -> (0, 0)
  line L140 (0, -20) -> (5, -20)
  line L141 (5, -20) -> (5, -40)
  line L142 (0, 0) -> (0, 20)
  line L143 (0, 0) -> (5, 0)
  line L144 (0, 20) -> (0, 40)
  line L145 (0, 20) -> (5, 20)
  line L146 (5, 20) -> (5, 0)
  line L147 (0, 40) -> (0, 60)
  line L148 (0, 40) -> (5, 40)
  line L149 (5, 40) -> (5, 20)
  line L150 (0, 60) -> (0, 80)
  line L151 (0, 60) -> (5, 60)
  line L152 (5, 60) -> (5, 40)
  line L153 (0, 80) -> (0, 100)
  line L154 (0, 80) -> (5, 80)
  line L155 (5, 80) -> (5, 60)
  line L156 (0, 100) -> (0, 120)
  line L157 (0, 100) -> (5, 100)
  line L158 (5, 100) -> (5, 80)
  line L159 (0, 120) -> (0, 140)
  line L160 (0, 120) -> (5, 120)
  line L161 (5, 120) -> (5, 100)
  line L162 (0, 140) -> (0, 160)
  line L163 (0, 140) -> (5, 140)
  line L164 (5, 140) -> (5, 120)
  line L165 (0, 160) -> (0, 180)
  line L166 (0, 160) -> (5, 160)
  line L167 (5, 160) -> (5, 140)
  line L168 (0, 180) -> (0, 200)
  line L169 (0, 180) -> (5, 180)
  line L170 (5, 180) -> (5, 160)
  line L171 (0, 200) -> (0, 220)
  line L172 (0, 200) -> (5, 200)
  line L173 (5, 200) -> (5, 180)
  line L174 (0, 220) -> (0, 240)
  line L175 (0, 220) -> (5, 220)
  line L176 (5, 220) -> (5, 200)
  line L177 (0, 240) -> (0, 260)
  line L178 (0, 240) -> (5, 240)
  line L179 (5, 240) -> (5, 220)
  line L180 (0, 260) -> (0, 280)
  line L181 (0, 260) -> (5, 260)
  line L182 (5, 260) -> (5, 240)
  line L183 (0, 280) -> (0, 300)
  line L184 (0, 280) -> (5, 280)
  line L185 (5, 280) -> (5, 260)
  line L186 (0, 300) -> (0, 320)
  line L187 (0, 300) -> (5, 300)
  line L188 (5, 300) -> (5, 280)
  line L189 (0, 320) -> (0, 340)
  line L190 (0, 320) -> (5, 320)
  line L191 (5, 320) -> (5, 300)
  line L192 (0, 340) -> (0, 360)
  line L193 (0, 340) -> (5, 340)
  line L194 (5, 340) -> (5, 320)
  line L195 (0, 360) -> (0, 380)
  line L196 (0, 360) -> (5, 360)
  line L197 (5, 360) -> (5, 340)
  line L198 (0, 380) -> (0, 400)
  line L199 (0, 380) -> (5, 380)
  line L200 (5, 380) -> (5, 360)
  line L201 (0, 400) -> (0, 420)
  line L202 (0, 400) -> (5, 400)
  line L203 (5, 400) -> (5, 380)
  line L204 (0, 420) -> (0, 440)
  line L205 (0, 420) -> (5, 420)
  line L206 (5, 420) -> (5, 400)
  line L207 (0, 440) -> (0, 460)
  line L208 (0, 440) -> (5, 440)
  line L209 (5, 440) -> (5, 420)
  line L210 (0, 460) -> (0, 480)
  line L211 (0, 460) -> (5, 460)
  line L212 (5, 460) -> (5, 440)
  line L213 (0, 480) -> (0, 500)
  line L214 (0, 480) -> (5, 480)
  line L215 (5, 480) -> (5, 460)
  line L216 (0, 500) -> (0, 520)
  line L217 (0, 500) -> (5, 500)
  line L218 (5, 500) -> (5, 480)
  line L219 (0, 520) -> (5, 520)
  line L220 (5, 520) -> (5, 500)
  line L221 (5, 0) -> (5, -20)
  line L222 (5, 520) -> (6, 520)
  line L223 (6, 520) -> (6, -520)
  line L224 (6, -520) -> (5, -520)
  line L225 (12.3, -9.25) -> (12.3, -10.75)
  line L226 (12.3, -10.75) -> (17.8, -10.75)
  line L227 (17.8, -10.75) -> (17.8, -11.25)
  line L228 (17.8, -11.25) -> (12.3, -11.25)
  line L229 (12.3, -11.25) -> (12.3, -12.75)
  line L230 (12.3, -12.75) -> (17.8, -12.75)
  line L231 (17.8, -12.75) -> (17.8, -13.25)
  line L232 (17.8, -13.25) -> (12.3, -13.25)
  line L233 (12.3, -13.25) -> (12.3, -14.75)
  line L234 (12.3, -14.75) -> (17.8, -14.75)
  line L235 (17.8, -14.75) -> (17.8, -15.25)
  line L236 (17.8, -15.25) -> (12.3, -15.25)
  line L237 (12.3, -15.25) -> (12.3, -16.75)
  line L238 (12.3, -16.75) -> (17.8, -16.75)
  line L239 (17.8, -16.75) -> (17.8, -17.25)
  line L240 (17.8, -17.25) -> (12.3, -17.25)
  line L241 (12.3, -17.25) -> (12.3, -18.75)
  line L242 (12.3, -18.75) -> (17.8, -18.75)
  line L243 (17.8, -18.75) -> (17.8, -19.25)
  line L244 (17.8, -19.25) -> (12.3, -19.25)
  line L245 (12.3, -19.25) -> (12.3, -20.75)
  line L246 (12.3, -20.75) -> (17.8, -20.75)
  line L247 (17.8, -20.75) -> (17.8, -21.25)
  line L248 (17.8, -21.25) -> (12.3, -21.25)
  line L249 (12.3, -21.25) -> (12.3, -22.75)
  line L250 (12.3, -22.75) -> (17.8, -22.75)
  line L251 (17.8, -22.75) -> (17.8, -23.25)
  line L252 (17.8, -23.25) -> (12.3, -23.25)
  line L253 (12.3, -23.25) -> (12.3, -24.75)
  line L254 (12.3, -24.75) -> (17.8, -24.75)
  line L255 (17.8, -24.75) -> (17.8, -25.25)
  line L256 (17.8, -25.25) -> (12.3, -25.25)
  line L257 (12.3, -25.25) -> (12.3, -26.75)
  line L258 (12.3, -26.75) -> (17.8, -26.75)
  line L259 (17.8, -26.75) -> (17.8, -27.25)
  line L260 (17.8, -27.25) -> (12.3, -27.25)
  line L261 (12.3, -27.25) -> (12.3, -28.75)
  line L262 (12.3, -28.75) -> (17.8, -28.75)
  line L263 (17.8, -28.75) -> (17.8, -29.25)
  line L264 (17.8, -29.25) -> (12.3, -29.25)
  line L265 (12.3, -29.25) -> (12.3, -30.75)
  line L266 (12.3, -30.75) -> (17.8, -30.75)
  line L267 (17.8, -30.75) -> (17.8, -31.25)
  line L268 (17.8, -31.25) -> (12.3, -31.25)
  line L269 (12.3, -31.25) -> (12.3, -32.75)
  line L270 (12.3, -32.75) -> (17.8, -32.75)
  line L271 (17.8, -32.75) -> (17.8, -33.25)
  line L272 (17.8, -33.25) -> (12.3, -33.25)
  line L273 (12.3, -33.25) -> (12.3, -34.75)
  line L274 (17.8, 51.25) -> (17.8, 50.75)
  line L275 (17.8, 50.75) -> (12.3, 50.75)
  line L276 (12.3, 50.75) -> (12.3, 49.25)
  line L277 (12.3, 49.25) -> (17.8, 49.25)
  line L278 (17.8, 49.25) -> (17.8, 48.75)
  line L279 (17.8, 48.75) -> (12.3, 48.75)
  line L280 (12.3, 48.75) -> (12.3, 47.25)
  line L281 (12.3, 47.25) -> (17.8, 47.25)
  line L282 (17.8, 47.25) -> (17.8, 46.75)
  line L283 (17.8, 46.75) -> (12.3, 46.75)
  line L284 (12.3, 46.75) -> (12.3, 45.25)
  line L285 (12.3, 45.25) -> (17.8, 45.25)
  line L286 (17.8, 45.25) -> (17.8, 44.75)
  line L287 (17.8, 44.75) -> (12.3, 44.75)
  line L288 (12.3, 44.75) -> (12.3, 43.25)
  line L289 (12.3, 43.25) -> (17.8, 43.25)
  line L290 (17.8, 43.25) -> (17.8, 42.75)
  line L291 (17.8, 42.75) -> (12.3, 42.75)
  line L292 (12.3, 42.75) -> (12.3, 41.25)
  line L293 (12.3, 41.25) -> (17.8, 41.25)
  line L294 (17.8, 41.25) -> (17.8, 40.75)
  line L295 (17.8, 40.75) -> (12.3, 40.75)
  line L296 (12.3, 40.75) -> (12.3, 39.25)
  line L297 (12.3, 39.25) -> (17.8, 39.25)
  line L298 (17.8, 39.25) -> (17.8, 38.75)
  line L299 (17.8, 38.75) -> (12.3, 38.75)
  line L300 (12.3, 38.75) -> (12.3, 37.25)
  line L301 (12.3, 37.25) -> (17.8, 37.25)
  line L302 (17.8, 37.25) -> (17.8, 36.75)
  line L303 (17.8, 36.75) -> (12.3, 36.75)
  line L304 (12.3, 36.75) -> (12.3, 35.25)
  line L305 (12.3, 35.25) -> (17.8, 35.25)
  line L306 (17.8, 35.25) -> (17.8, 34.75)
  line L307 (17.8, 34.75) -> (12.3, 34.75)
  line L308 (12.3, 34.75) -> (12.3, 33.25)
  line L309 (12.3, 33.25) -> (17.8, 33.25)
  line L310 (17.8, 33.25) -> (17.8, 32.75)
  line L311 (17.8, 32.75) -> (12.3, 32.75)
  line L312 (12.3, 32.75) -> (12.3, 31.25)
  line L313 (12.3, 31.25) -> (17.8, 31.25)
  line L314 (17.8, 31.25) -> (17.8, 30.75)
  line L315 (17.8, 30.75) -> (12.3, 30.75)
  line L316 (12.3, 30.75) -> (12.3, 29.25)
  line L317 (12.3, 29.25) -> (17.8, 29.25)
  line L318 (17.8, 29.25) -> (17.8, 28.75)
  line L319 (17.8, 28.75) -> (12.3, 28.75)
  line L320 (12.3, 28.75) -> (12.3, 27.25)
  line L321 (12.3, 27.25) -> (17.8, 27.25)
  line L322 (17.8, 27.25) -> (17.8, 26.75)
  line L323 (17.8, 26.75) -> (12.3, 26.75)
  line L324 (12.3, 26.75) -> (12.3, 25.25)
  line L325 (12.3, 25.25) -> (17.8, 25.25)
  line L326 (17.8, 25.25) -> (17.8, 24.75)
  line L327 (17.8, 24.75) -> (12.3, 24.75)
  line L328 (12.3, 24.75) -> (12.3, 23.25)
  line L329 (12.3, 23.25) -> (17.8, 23.25)
  line L330 (17.8, 23.25) -> (17.8, 22.75)
  line L331 (17.8, 22.75) -> (12.3, 22.75)
  line L332 (12.3, 22.75) -> (12.3, 21.25)
  line L333 (12.3, 21.25) -> (17.8, 21.25)
  line L334 (17.8, 21.25) -> (17.8, 20.75)
  line L335 (17.8, 20.75) -> (12.3, 20.75)
  line L336 (12.3, 20.75) -> (12.3, 19.25)
  line L337 (12.3, 19.25) -> (17.8, 19.25)
  line L338 (17.8, 19.25) -> (17.8, 18.75)
  line L339 (17.8, 18.75) -> (12.3, 18.75)
  line L340 (12.3, 18.75) -> (12.3, 17.25)
  line L341 (12.3, 17.25) -> (17.8, 17.25)
  line L342 (17.8, 17.25) -> (17.8, 16.75)
  line L343 (17.8, 16.75) -> (12.3, 16.75)
  line L344 (12.3, 16.75) -> (12.3, 15.25)
  line L345 (12.3, 15.25) -> (17.8, 15.25)
  line L346 (17.8, 15.25) -> (17.8, 14.75)
  line L347 (17.8, 14.75) -> (12.3, 14.75)
  line L348 (12.3, 14.75) -> (12.3, 13.25)
  line L349 (12.3, 13.25) -> (17.8, 13.25)
  line L350 (17.8, 13.25) -> (17.8, 12.75)
  line L351 (17.8, 12.75) -> (12.3, 12.75)
  line L352 (12.3, 12.75) -> (12.3, 11.25)
  line L353 (12.3, 11.25) -> (17.8, 11.25)
  line L354 (17.8, 11.25) -> (17.8, 10.75)
  line L355 (17.8, 10.75) -> (12.3, 10.75)
  line L356 (12.3, 10.75) -> (12.3, 9.25)
  line L357 (12.3, 9.25) -> (17.8, 9.25)
  line L358 (17.8, 9.25) -> (17.8, 8.75)
  line L359 (17.8, 8.75) -> (12.3, 8.75)
  line L360 (12.3, 8.75) -> (12.3, 7.25)
  line L361 (12.3, 7.25) -> (17.8, 7.25)
  line L362 (17.8, 7.25) -> (17.8, 6.75)
  line L363 (17.8, 6.75) -> (12.3, 6.75)
  line L364 (12.3, 6.75) -> (12.3, 5.25)
  line L365 (12.3, 5.25) -> (17.8, 5.25)
  line L366 (17.8, 5.25) -> (17.8, 4.75)
  line L367 (17.8, 4.75) -> (12.3, 4.75)
  line L368 (12.3, 4.75) -> (12.3, 3.25)
  line L369 (12.3, 3.25) -> (17.8, 3.25)
  line L370 (17.8, 3.25) -> (17.8, 2.75)
  line L371 (17.8, 2.75) -> (12.3, 2.75)
  line L372 (12.3, 2.75) -> (12.3, 1.25)
  line L373 (12.3, 1.25) -> (17.8, 1.25)
  line L374 (17.8, 1.25) -> (17.8, 0.75)
  line L375 (17.8, 0.75) -> (12.3, 0.75)
  line L376 (12.3, 0.75) -> (12.3, -0.75)
  line L377 (12.3, -0.75) -> (17.8, -0.75)
  line L378 (17.8, -0.75) -> (17.8, -1.25)
  line L379 (17.8, -1.25) -> (12.3, -1.25)
  line L380 (12.3, -1.25) -> (12.3, -2.75)
  line L381 (12.3, -2.75) -> (17.8, -2.75)
  line L382 (17.8, -2.75) -> (17.8, -3.25)
  line L383 (17.8, -3.25) -> (12.3, -3.25)
  line L384 (12.3, -3.25) -> (12.3, -4.75)
  line L385 (12.3, -4.75) -> (17.8, -4.75)
  line L386 (17.8, -4.75) -> (17.8, -5.25)
  line L387 (17.8, -5.25) -> (12.3, -5.25)
  line L388 (12.3, -5.25) -> (12.3, -6.75)
  line L389 (12.3, -6.75) -> (17.8, -6.75)
  line L390 (17.8, -6.75) -> (17.8, -7.25)
  line L391 (17.8, -7.25) -> (12.3, -7.25)
  line L392 (12.3, -7.25) -> (12.3, -8.75)
  line L393 (12.3, -8.75) -> (17.8, -8.75)
  line L394 (17.8, -8.75) -> (17.8, -9.25)
  line L395 (17.8, -9.25) -> (12.3, -9.25)
  line L396 (10.5, 11) -> (10.5, 9)
  line L397 (11.5, -30) -> (11.5, 50)
  line L398 (12.3, -34.75) -> (12.3, -35)
  line L399 (12.3, -35) -> (11.5, -35)
  line L400 (11.5, 50) -> (11.5, 51.25)
  line L401 (11.5, 51.25) -> (11.5, 51.4522)
  line L402 (17.8, 51.4522) -> (17.8, 51.25)
  line L403 (6.5, -35) -> (9, -35)
  line L404 (6.5, -35) -> (6.5, -38)
  line L405 (9, -35) -> (9.1, -35)
  line L406 (12.3, -35) -> (12.4, -35)
  line L407 (12.4, -35) -> (12.4, -33.25)
  line L408 (17.8, -33.25) -> (17.8, -38)
  line L409 (6.5, -38) -> (17.8, -38)
  line L410 (10.5, 50) -> (11.4, 50)
  line L411 (11.4, 50) -> (11.4, 51.4522)
  line L412 (11.4, 51.4522) -> (11.5, 51.4522)
  line L413 (11.5, 51.4522) -> (17.8, 51.4522)
  line L414 (6.5, 55) -> (17.8, 55)
  line L415 (17.8, 55) -> (17.8, 51.4522)
  line L416 (10.5, -30) -> (10.7, -30)
  line L417 (10.7, -30) -> (10.7, -33)
  line L418 (10.7, -33) -> (10.7, -35)
  line L419 (10.7, -35) -> (9, -35)
  line L420 (11.5, -35) -> (10.7, -35)
  dimension "d6" = 3
  dimension "d7" = 0.1
  dimension "d12" = 0.9
  dimension "d14" = 0.2
  constraint parallel L397 L400
  constraint perpendicular L403 L404
  constraint horizontal L406
  constraint coincident L272 L407.end
  constraint perpendicular L272 L407
  constraint perpendicular L410 L411
  constraint perpendicular L401 L412
  constraint parallel L412 L413
  constraint perpendicular L402 L414
  constraint perpendicular L413 L415
  constraint perpendicular L53 L416
  constraint parallel L417 L418
  measures "d6" distance of L52.start L404.end
  measures "d7" distance of L398.end L406.end
  measures "d12" distance of L39.end L410.end
  measures "d14" distance of L7.start L416.end
revolve "Revolve9" add sketch "motor_base_geometry" angle 360 about axis through (0, 0, 20) along (0, 0, -1) contours L51 L225 L226 L227 L228 L229 L230 L231 L232 L233 L234 L235 L236 L237 L238 L239 L240 L241 L242 L243 L244 L245 L246 L247 L248 L249 L250 L251 L252 L253 L254 L255 L256 L257 L258 L259 L260 L261 L262 L263 L264 L265 L266 L267 L268 L269 L270 L271 L272 L273 L274 L275 L276 L277 L278 L279 L280 L281 L282 L283 L284 L285 L286 L287 L288 L289 L290 L291 L292 L293 L294 L295 L296 L297 L298 L299 L300 L301 L302 L303 L304 L305 L306 L307 L308 L309 L310 L311 L312 L313 L314 L315 L316 L317 L318 L319 L320 L321 L322 L323 L324 L325 L326 L327 L328 L329 L330 L331 L332 L333 L334 L335 L336 L337 L338 L339 L340 L341 L342 L343 L344 L345 L346 L347 L348 L349 L350 L351 L352 L353 L354 L355 L356 L357 L358 L359 L360 L361 L362 L363 L364 L365 L366 L367 L368 L369 L370 L371 L372 L373 L374 L375 L376 L377 L378 L379 L380 L381 L382 L383 L384 L385 L386 L387 L388 L389 L390 L391 L392 L393 L394 L395 L397 L398 L399 L400 L401 L402 L413
named bodies: "Heat Sink"

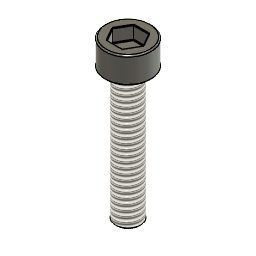
design "m2 x 10"
Autodesk Fusion 360 part; units mm, degrees
sketch "main" plane through (0, 0, 0) normal (0, 1, 0) x (1, 0, 0)
  circle A0 centre (0, 0) radius 1
  circle A1 centre (0, 0) radius 1.75
  dimension "d1" = 2
  dimension "d2" = 3.5
  constraint coincident A0.centre A1.centre
  constraint concentric A0 A1
  measures "d1" diameter of A0
  measures "d2" diameter of A1
extrude "Extrude1" add sketch "main" along normal blind 2 contours A0 | A1
extrude "Extrude2" add sketch "main" against normal blind 10 contours A0
fillet "Fillet1" radius 0.1 4 edges at (-0.9323, 0, 0.3616) (-1.6316, 2, 0.6328) (-1.6316, 0, 0.6328) (-0.9323, -10, -0.3616)
thread "Thread1" "ISO Metric profile 2.0 M2x0.4 M2x0.4 6g" major diameter 1.9335 minor diameter 1.478 pitch 0.4 angle 60 resizes the face on face at (0.995, -6.6333, 0.0996)
sketch "m2" plane through (0, 2, 0) normal (0, 1, 0) x (-1, 0, 0)
  circle A0 centre (0, 0) radius 1.65
  line L0 (-0.5774, 1) -> (-1.1547, 0)
  line L1 (-1.1547, 0) -> (-0.5774, -1)
  line L2 (-0.5774, -1) -> (0.5774, -1)
  line L3 (0.5774, -1) -> (1.1547, 0)
  line L4 (1.1547, 0) -> (0.5774, 1)
  line L5 (0.5774, 1) -> (-0.5774, 1)
  dimension "d11" = 1
  constraint coincident A0.centre origin
  measures "d11" distance of A0.centre L5
extrude "Extrude3" cut sketch "m2" against normal blind 1 contours L0 L1 L2 L3 L4 L5
chamfer "Chamfer1" distance 0.05 angle 45 12 edges at (-0.866, 1, 0.5) (0, 1, 1) (0.866, 1, 0.5) (0.866, 1, -0.5) (0, 1, -1) (-0.866, 1, -0.5) (-0.866, 2, 0.5) (0, 2, 1) (0.866, 2, 0.5) (0.866, 2, -0.5) (0, 2, -1) (-0.866, 2, -0.5)
named bodies: "main"

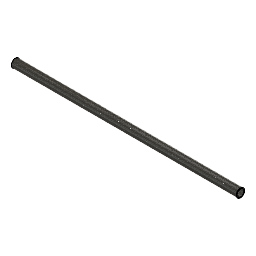
design "Carbon fibre pipe"
Autodesk Fusion 360 part; units mm, degrees
sketch "Sketch1" plane through (0, 0, 0) normal (1, 0, 0) x (0, 0, -1)
  circle A0 centre (0, 0) radius 5
  circle A1 centre (0, 0) radius 6
  dimension "d1" = 10
  dimension "d2" = 12
  constraint coincident A0.centre A1.centre
  measures "d1" diameter of A0
  measures "d2" diameter of A1
extrude "Extrude1" add sketch "Sketch1" along normal blind 320

design "M3 x 5mm"
Autodesk Fusion 360 part; units mm, degrees
sketch "main" plane through (0, 0, 0) normal (0, 1, 0) x (1, 0, 0)
  circle A0 centre (0, 0) radius 1.5
  circle A1 centre (0, 0) radius 2.6
  dimension "d1" = 3
  dimension "d2" = 5.2
  constraint coincident A0.centre A1.centre
  measures "d1" diameter of A0
  measures "d2" diameter of A1
extrude "Extrude1" add sketch "main" along normal blind 3 contours A0 | A1
extrude "Extrude2" add sketch "main" against normal blind 5 contours A0
fillet "Fillet1" radius 0.1 1 edges at (-1.3985, -5, -0.5424)
fillet "Fillet2" radius 0.1 3 edges at (-1.3985, 0, 0.5424) (-2.4241, 0, 0.9402) (-2.4241, 3, 0.9402)
thread "Thread1" "ISO Metric profile 3.0 M3x0.5 M3x0.5 6g" major diameter 2.927 minor diameter 2.3555 pitch 0.5 angle 60 resizes the face on face at (1.4981, -3.3, 0.0748)
sketch "3mm hex" plane through (0, 3, 0) normal (0, 1, 0) x (-1, 0, 0)
  circle A0 centre (0, 0) radius 2.5
  line L0 (0.866, -1.5) -> (1.7321, 0)
  line L1 (1.7321, 0) -> (0.866, 1.5)
  line L2 (0.866, 1.5) -> (-0.866, 1.5)
  line L3 (-0.866, 1.5) -> (-1.7321, 0)
  line L4 (-1.7321, 0) -> (-0.866, -1.5)
  line L5 (-0.866, -1.5) -> (0.866, -1.5)
  dimension "d13" = 1.5
  constraint coincident A0.centre origin
  measures "d13" distance of A0.centre L5
extrude "Extrude3" cut sketch "3mm hex" against normal blind 2 contours L0 L1 L2 L3 L4 L5
chamfer "Chamfer1" distance 0.1 angle 45 12 edges at (-1.299, 1, -0.75) (0, 1, -1.5) (1.299, 1, -0.75) (1.299, 1, 0.75) (0, 1, 1.5) (-1.299, 1, 0.75) (0, 3, 1.5) (-1.299, 3, 0.75) (-1.299, 3, -0.75) (0, 3, -1.5) (1.299, 3, -0.75) (1.299, 3, 0.75)
equation "d13 = ( 3 / 2 ) * 1 mm"

design "m2 x 6"
Autodesk Fusion 360 part; units mm, degrees
sketch "main" plane through (0, 0, 0) normal (0, 1, 0) x (1, 0, 0)
  circle A0 centre (0, 0) radius 1
  circle A1 centre (0, 0) radius 1.75
  dimension "d1" = 2
  dimension "d2" = 3.5
  constraint coincident A0.centre A1.centre
  constraint concentric A0 A1
  measures "d1" diameter of A0
  measures "d2" diameter of A1
extrude "Extrude1" add sketch "main" along normal blind 2 contours A0 | A1
extrude "Extrude2" add sketch "main" against normal blind 6 contours A0
fillet "Fillet1" radius 0.1 4 edges at (-0.9323, 0, 0.3616) (-1.6316, 2, 0.6328) (-1.6316, 0, 0.6328) (-0.9323, -6, -0.3616)
thread "Thread1" "ISO Metric profile 2.0 M2x0.4 M2x0.4 6g" major diameter 1.9335 minor diameter 1.478 pitch 0.4 angle 60 resizes the face on face at (0.995, -3.9667, 0.0996)
sketch "m2" plane through (0, 2, 0) normal (0, 1, 0) x (-1, 0, 0)
  circle A0 centre (0, 0) radius 1.65
  line L0 (-0.5774, 1) -> (-1.1547, 0)
  line L1 (-1.1547, 0) -> (-0.5774, -1)
  line L2 (-0.5774, -1) -> (0.5774, -1)
  line L3 (0.5774, -1) -> (1.1547, 0)
  line L4 (1.1547, 0) -> (0.5774, 1)
  line L5 (0.5774, 1) -> (-0.5774, 1)
  dimension "d11" = 1
  constraint coincident A0.centre origin
  measures "d11" distance of A0.centre L5
extrude "Extrude3" cut sketch "m2" against normal blind 1 contours L0 L1 L2 L3 L4 L5
chamfer "Chamfer1" distance 0.05 angle 45 12 edges at (-0.866, 1, 0.5) (0, 1, 1) (0.866, 1, 0.5) (0.866, 1, -0.5) (0, 1, -1) (-0.866, 1, -0.5) (-0.866, 2, 0.5) (0, 2, 1) (0.866, 2, 0.5) (0.866, 2, -0.5) (0, 2, -1) (-0.866, 2, -0.5)

design "linear scale insert"
Autodesk Fusion 360 part; units mm, degrees